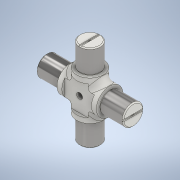
# Autodesk Inventor part: Part10.Universal Joint Cross
Saved by Autodesk Inventor 2022.2 (Build 262287010, 287A)
## iProperties
Created: 2022-12-06
Part Number: Part10.Universal Joint Cross
Material: Steel, Wrought
Document SubType Name: Modeling
Designer: User
Mass: 486.762 g
Surface Area: 140.206 cm^2
Volume: 62.0078 cm^3
Density: 7.85 g/cm^3
Appearance: Steel
Author: User
Autodesk Inventor part; units mm, degrees
ref_plane "YZ Plane" through (0, 0, 0) normal (1, 0, 0) x (0, 1, 0)
ref_plane "XZ Plane" through (0, 0, 0) normal (0, 1, 0) x (-1, 0, 0)
sketch "Sketch1" plane through (0, 0, 0) normal (0, 0, 1) x (1, 0, 0)
  line L0 (20, 0) -> (-20, 0)
  line L1 (-20, 0) -> (-20, 13.5)
  line L2 (-20, 13.5) -> (20, 13.5)
  line L3 (20, 13.5) -> (20, 0)
  point P0 (0, 0)
  point P1 (0, 0)
  dimension "d0" = 27
  dimension "d1" = 40
  constraints: 8 end point, 2 parallel, 1 coincident, 1 horizontal, 1 midpoint, 1 perpendicular
  measures "d0" diameter of L2 L0
  measures "d1" distance of L1.end L2.end
revolve "Revolution1" add sketch "Sketch1" angle 360 about axis through (20, 0, 0) along (-1, 0, 0)
sketch "Sketch2" plane through (0, 0, 0) normal (0, 0, 1) x (1, 0, 0)
  line L0 (-13.5, 20) -> (0, 20)
  line L1 (0, 20) -> (0, -20)
  line L2 (0, -20) -> (-13.5, -20)
  line L3 (-13.5, -20) -> (-13.5, 20)
  point P0 (0, 0)
  point P1 (0, 0)
  dimension "d3" = 27
  dimension "d4" = 40
  constraints: 8 end point, 2 parallel, 1 coincident, 1 horizontal, 1 midpoint, 1 perpendicular
  measures "d3" diameter of L3 L1
  measures "d4" distance between parallel lines of L2 L0
revolve "Revolution2" add sketch "Sketch2" angle 360 about axis through (0, 20, 0) along (0, -1, 0)
fillet "Fillet1" radius 6 7 edges at (9.5459, 9.5459, -9.5459) (13.5, -13.5, 0) (9.5459, 9.5459, 9.5459) (-9.5459, 9.5459, -9.5459) (-9.5459, 9.5459, 9.5459) (-9.5459, -9.5459, 9.5459) (-9.5459, -9.5459, -9.5459)
sketch "Sketch3" plane through (0, 0, 0) normal (0, 0, 1) x (1, 0, 0)
  line L0 (0, 0) -> (0, 0) projected
  line L1 (0, 0) -> (0, 0) projected
  line L2 (-20, -13.5) -> (-20, 13.5) projected
  line L3 (-20, 10) -> (-21, 10)
  line L4 (-21, 10) -> (-21, 10.5)
  line L5 (-21, 10.5) -> (-44, 10.5)
  line L6 (-44, 10.5) -> (-44, 0)
  line L7 (-44, 0) -> (-20, 0)
  line L8 (-20, 0) -> (-20, 10)
  point P0 (0, 0)
  point P1 (-20.5, 10)
  dimension "d7" = 21
  dimension "d8" = 44
  dimension "d9" = 20
  dimension "d10" = 1
  constraints: 12 end point, 3 perpendicular, 2 midpoint, 1 collinear, 1 horizontal, 1 point on line
  measures "d7" diameter of L5 L7
  measures "d8" distance from line of point (0, 0) L6
  measures "d9" diameter of point (-20.5, 10) L7
  measures "d10" distance of L3.start L3.end
revolve "Revolution3" add sketch "Sketch3" angle 360 about axis through (-44, 0, 0) along (1, 0, 0)
chamfer "Chamfer1" distance 1 angle 45 1 edges at (-44, -10.5, 0)
sketch "Sketch4" plane through (0, 0, 0) normal (0, 0, 1) x (1, 0, 0)
  line L0 (-44, 1) -> (-43, 1)
  line L1 (-43, 1) -> (-43, -1)
  line L2 (-43, -1) -> (-44, -1)
  line L3 (-44, -1) -> (-44, 1)
  line L4 (-44, -9.5) -> (-44, 9.5) construction
  point P0 (0, 0)
  point P1 (-44, 0)
  dimension "d15" = 1
  dimension "d16" = 2
  constraints: 8 end point, 2 midpoint, 2 parallel, 1 horizontal, 1 perpendicular
  measures "d15" distance of L1.end L2.end
  measures "d16" distance of L0.end L1.end
extrude "Extrusion1" cut sketch "Sketch4" along normal through all both and the other way through all
pattern_circular "Circular Pattern1" count 4 over 360 about axis through (0, 0, -10) along (0, 0, 1) of "Revolution3", "Chamfer1", "Extrusion1"
ref_plane "Work Plane1" through (0, 0, 10.5) normal (0, 0, 1) x (1, 0, 0)
sketch "Sketch5" plane through (0, 0, 10.5) normal (0, 0, 1) x (1, 0, 0)
  line L0 (-15, -15) -> (15, -15)
  line L1 (15, -15) -> (15, 15)
  line L2 (15, 15) -> (-15, 15)
  line L3 (-15, 15) -> (-15, -15)
  line L4 (-15, -15) -> (15, 15) construction
  line L5 (15, -15) -> (-15, 15) construction
  point P0 (0, 0)
  dimension "d23" = 30
  dimension "d24" = 30
  constraints: 12 end point, 2 midpoint, 2 parallel, 1 horizontal, 1 perpendicular
  measures "d23" distance of L2.end L1.end
  measures "d24" distance of L1.end L0.end
extrude "Extrusion2" cut sketch "Sketch5" along normal through all
mirror "Mirror1" about plane through (0, 0, 0) normal (0, 0, 1) of "Extrusion2"
sketch "Sketch6" plane through (0, 0, 10.5) normal (0, 0, 1) x (1, 0, 0)
  point P0 (0, 0)
hole "Hole1" at (0, 0, 10.5) direction (0, 0, -1) diameter 2 end through all counterbore diameter 6 counterbore depth 5
sketch "Sketch7" plane through (0, 43, 0) normal (0, 1, 0) x (1, 0, 0)
  arc A0 (-1, -10.4523) -> (1, -10.4523) centre (0, 0) ccw projected
  point P0 (0, 0)
  constraints: 1 coincident
hole "Hole2" at (0, 43, 0) direction (0, -1, 0) diameter 2 end through all
sketch "Sketch8" plane through (43, 0, 0) normal (1, 0, 0) x (0, 0, -1)
  arc A0 (-10.4523, 1) -> (-10.4523, -1) centre (0, 0) ccw projected
  point P0 (0, 0)
  constraints: 1 coincident
hole "Hole3" at (43, 0, 0) direction (-1, 0, 0) diameter 2 end through all
equation "\"d3\" = d0"
equation "\"d4\" = d1"
body "Solid1"
